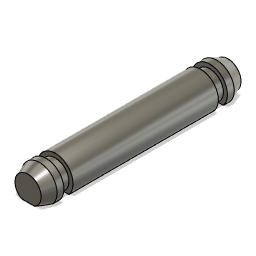
Pins Shrt (30mm) v1 (Autodesk Fusion 360 design; units mm, degrees)
Autodesk Fusion 360 part; units mm, degrees
sketch "Sketch1" plane through (0, 0, 0) normal (0, 0, 1) x (1, 0, 0)
  line L0 (0, 0) -> (5.9867, 0)
  arc A0 (5.9867, 0) -> (0, 0) centre (2.9933, 2.5) ccw
  arc A1 (4.6516, 0) -> (1.335, 0) centre (2.9933, 2.5) ccw
  arc A2 (17.1516, 0) -> (13.835, 0) centre (15.4933, 2.5) ccw
  line L1 (12.5, 0) -> (18.4867, 0)
  arc A3 (18.4867, 0) -> (12.5, 0) centre (15.4933, 2.5) ccw
  arc A4 (29.6516, 0) -> (26.335, 0) centre (27.9933, 2.5) ccw
  line L2 (25, 0) -> (30.9867, 0)
  arc A5 (30.9867, 0) -> (25, 0) centre (27.9933, 2.5) ccw
  point P0 (12.5, 0)
  point P1 (25, 0)
  dimension "d1" = 3.9
  dimension "d2" = 2.5
  dimension "d13" = 6
  dimension "d16" = 25
  dimension "d17" = 0
  constraint coincident L0.start A0.end
  constraint horizontal L0
  constraint concentric A0 A1
  constraint coincident L0 A1.end
  constraint coincident L0 A1.start
  measures "d1" radius of A0
  measures "d2" distance of L0 A0.centre
  measures "d13" diameter of A1
extrude "Extrude1" add sketch "Sketch1" along normal blind 102 contours L0 A0 A1 | L0 A1 makes body 1
extrude "Extrude2" cut sketch "Sketch1" against normal blind 2 from surface at 6 contours L0 A0 A1 bodies 1
ref_plane "WorkPlane1" through (2.9933, 3.9289, 51) normal (0, 0, 1) x (1, 0, 0)
mirror "Mirror1" about plane through (2.9933, 3.9289, 51) normal (0, 0, 1) of "Extrude2"
extrude "Extrude3" add sketch "Sketch1" along normal blind 44 separate body contours A2 L1 | A2 L1 A3 makes body 2
extrude "Extrude4" cut sketch "Sketch1" against normal blind 2 from surface at 6 contours A2 L1 A3 bodies 2
ref_plane "WorkPlane2" through (15.4933, 3.9289, 22) normal (0, 0, 1) x (1, 0, 0)
mirror "Mirror2" about plane through (15.4933, 3.9289, 22) normal (0, 0, 1) of "Extrude4"
chamfer "Chamfer3" distance 2.5 distance2 1 1 edges at (15.4933, 6.4, 0) measured on face at (12.3817, 0.1488, 2.6667) on bodies 1 2
chamfer "Chamfer3" distance 2.5 distance2 1 1 edges at (2.9933, 6.4, 0) measured on face at (-0.1183, 0.1488, 2.6667) on bodies 1 2
chamfer "Chamfer3" distance 1 distance2 2.5 2 edges at (15.4933, 6.4, 44) (2.9933, 6.4, 102) measured on face at (16.772, 1.0681, 44) measured on face at (3.5688, 2.2017, 102) on bodies 1 2
hidden bodies 1
equation "d7 = Long_Pin + End_Thickness * 2"
equation "C_Clip_Thickness = 2 mm"
equation "End_Thickness = 4 mm + C_Clip_Thickness"
equation "Long_Pin = 90 mm"
equation "Short_Pin = 32 mm"
equation "d18 = End_Thickness"
equation "d19 = -C_Clip_Thickness"
equation "d25 = Short_Pin + End_Thickness * 2"
equation "d27 = End_Thickness"
equation "d28 = -C_Clip_Thickness"
